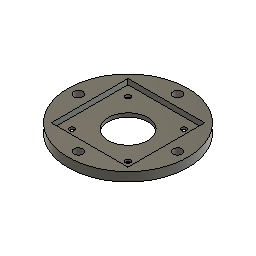
Nema17_clamping_part1 (Autodesk Fusion 360 design; units mm, degrees)
part number: 2025-04-27-14-45-54-431
Autodesk Fusion 360 part; units mm, degrees
sketch "Sketch1" plane through (0, 0, 0) normal (0, 1, 0) x (1, 0, 0)
  circle A0 centre (0, 0) radius 11
  circle A1 centre (15.5, 15.5) radius 1.5
  circle A2 centre (-15.5, 15.5) radius 1.5
  circle A3 centre (-15.5, -15.5) radius 1.5
  circle A4 centre (15.5, -15.5) radius 1.5
  circle A5 centre (0, 0) radius 33.1
  circle A6 centre (0, 27.5) radius 2.5
  circle A7 centre (-27.5, 0) radius 2.5
  circle A8 centre (0, -27.5) radius 2.5
  circle A9 centre (27.5, 0) radius 2.5
  dimension "d1" = 22
  dimension "d2" = 3
  dimension "d3" = 15.5
  dimension "d5" = 360
  dimension "d6" = 66.2
  dimension "d7" = 5
  dimension "d8" = 27.5
  dimension "d10" = 360
  constraint coincident A0.centre A5.centre
  measures "d1" diameter of A0
  measures "d2" diameter of A1
  measures "d3" horizontal distance of A0.centre A1.centre
  measures "d6" diameter of A5
  measures "d7" diameter of A6
  measures "d8" distance of A0.centre A6.centre
extrude "Extrude1" add sketch "Sketch1" along normal blind 2
sketch "Sketch2" plane through (0, 2, 0) normal (0, 1, 0) x (-1, 0, 0)
  circle A0 centre (15.5, 15.5) radius 1.5
  circle A1 centre (0, 27.5) radius 2.5
  circle A2 centre (-15.5, -15.5) radius 1.5
  circle A3 centre (-15.5, 15.5) radius 1.5
  circle A4 centre (0, -27.5) radius 2.5
  circle A5 centre (0, 0) radius 11
  circle A6 centre (27.5, 0) radius 2.5
  circle A7 centre (15.5, -15.5) radius 1.5
  circle A8 centre (-27.5, 0) radius 2.5
  circle A9 centre (0, 0) radius 33.1
  line L0 (21.25, -21.25) -> (-21.25, -21.25)
  line L1 (-21.25, -21.25) -> (-21.25, 21.25)
  line L2 (-21.25, 21.25) -> (21.25, 21.25)
  line L3 (21.25, 21.25) -> (21.25, -21.25)
  line L4 (21.25, -21.25) -> (-21.25, 21.25) construction
  line L5 (-21.25, -21.25) -> (21.25, 21.25) construction
  dimension "d13" = 42.5
  dimension "d14" = 42.5
  constraint horizontal L0
  constraint perpendicular L0 L1
  constraint parallel L0 L2
  constraint parallel L1 L3
  constraint coincident L4 A5.centre
  constraint coincident L5 A5.centre
  constraint coincident A5.centre A9.centre
  measures "d13" distance of L1.end L2.end
  measures "d14" distance of L0.end L1.end
extrude "Extrude2" add sketch "Sketch2" along normal blind 3 contours A9
chamfer "Chamfer1" distance 0.75 angle 45 4 edges at (14.1015, 0, 14.9576) (14.1015, 0, -16.0424) (-16.8985, 0, -16.0424) (-16.8985, 0, 14.9576)
chamfer "Chamfer2" distance 1.5 angle 45 4 edges at (-2.3308, 0, 26.596) (25.1692, 0, -0.904) (-2.3308, 0, -28.404) (-29.8308, 0, -0.904)
